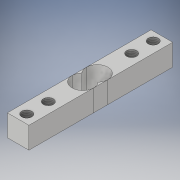
# Autodesk Inventor part: Load cell
Saved by Autodesk Inventor 2019 (Build 230136000, 136)
## iProperties
Created: 2021-03-05
Part Number: Load cell
Material: Generic
Document SubType Name: Modeling
Designer: User
Density: 1 g/cm^3
Appearance: Default
Author: User
Autodesk Inventor part; units mm, degrees
ref_plane "YZ Plane" through (0, 0, 0) normal (1, 0, 0) x (0, 1, 0)
ref_plane "XZ Plane" through (0, 0, 0) normal (0, 1, 0) x (-1, 0, 0)
ref_plane "XY Plane" through (0, 0, 0) normal (0, 0, 1) x (1, 0, 0)
sketch "Sketch2" plane through (0, 0, 0) normal (0, 1, 0) x (-1, 0, 0)
  arc A0 (5.5902, -5) -> (-5.5902, -5) centre (0, 0) ccw
  arc A1 (-5.5902, -5) -> (5.5902, -5) centre (0, -10) ccw
  line L0 (7.5, 45) -> (-7.5, 45)
  line L1 (-7.5, 45) -> (-7.5, -55)
  line L2 (-7.5, -55) -> (7.5, -55)
  line L3 (7.5, -55) -> (7.5, 45)
  dimension "d0" = 15
  dimension "d1" = 15
  dimension "d2" = 10
  dimension "d3" = 15
  dimension "d4" = 7.5
  dimension "d5" = 100
  dimension "d6" = 50
  dimension "d7" = 55
  constraints: 8 end point, 4 point on circle, 2 centre point, 2 parallel, 1 coincident, 1 horizontal, 1 perpendicular
  measures "d0" diameter of A0
  measures "d1" diameter of A1
  measures "d2" distance of A1.centre point (0, 0)
  measures "d3" distance between parallel lines of L1 L3
  measures "d4" distance from line of L3 point (0, 0)
  measures "d5" distance between parallel lines of L2 L0
  measures "d6" distance from line of L2 A0.start
  measures "d7" distance from line of A1.centre L0
extrude "Extrusion1" add sketch "Sketch2" along normal mid plane 15 contours A0 L3 A1 | A0 L1 L0 L3 | L3 L2 L1 A1 | A0 A1 L1
sketch "Sketch3" plane through (0, -7.5, 0) normal (0, -1, 0) x (1, 0, 0)
  circle A0 centre (0, -49) radius 3.5
  circle A1 centre (0, -34) radius 3.5
  line L0 (7.5, -55) -> (7.5, -10) projected
  line L1 (-7.5, -55) -> (7.5, -55) projected
  circle A2 centre (0, 24) radius 3.5
  circle A3 centre (0, 39) radius 3.5
  line L2 (7.5, 45) -> (-7.5, 45) projected
  point P0 (0, 0)
  dimension "d10" = 7
  dimension "d11" = 7
  dimension "d12" = 15
  dimension "d13" = 7.5
  dimension "d14" = 6
  dimension "d15" = 21
  dimension "d16" = 7
  dimension "d17" = 7
  dimension "d18" = 15
  dimension "d19" = 6
  dimension "d20" = 7.5
  dimension "d21" = 21
  constraints: 4 centre point
  measures "d10" diameter of A0
  measures "d11" diameter of A1
  measures "d12" distance of A1.centre A0.centre
  measures "d13" distance from line of A1.centre L0
  measures "d14" distance from line of A0.centre L1
  measures "d15" distance from line of A1.centre L1
  measures "d16" diameter of A2
  measures "d17" diameter of A3
  measures "d18" distance of A2.centre A3.centre
  measures "d19" distance from line of A3.centre L2
  measures "d20" distance from line of A3.centre L0
  measures "d21" distance from line of A2.centre L2
extrude "Extrusion2" cut sketch "Sketch3" against normal blind 15
thread "Thread1" size "M7x1" class "6H" standard "ANSI Metric M Profile" full length
thread "Thread2" size "M7x1" class "6H" standard "ANSI Metric M Profile" full length
thread "Thread3" size "M7x1" class "6H" standard "ANSI Metric M Profile" full length
thread "Thread4" size "M7x1" class "6H" standard "ANSI Metric M Profile" full length
body "Solid1"
